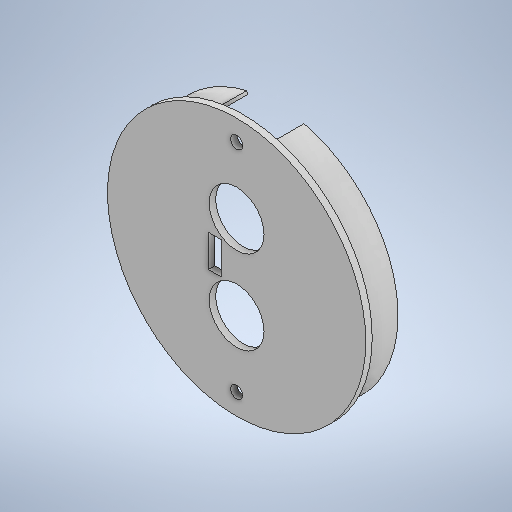
# Autodesk Inventor part: lid
Saved by Autodesk Inventor 2025.3 (Build 293356000, 356)
## iProperties
Created: 2025-04-18
Part Number: lid
Material: Generic
Document SubType Name: Modeling
Designer: Owner
Density: 1 g/cm^3
Appearance: Default
Author: Owner
Autodesk Inventor part; units mm, degrees
ref_plane "YZ Plane" through (0, 0, 0) normal (1, 0, 0) x (0, 1, 0)
ref_plane "XZ Plane" through (0, 0, 0) normal (0, 1, 0) x (-1, 0, 0)
ref_plane "XY Plane" through (0, 0, 0) normal (0, 0, 1) x (1, 0, 0)
sketch "Sketch1" plane through (0, 0, 0) normal (0, 0, 1) x (1, 0, 0)
  arc A0 (8.8755, -70.449) -> (8.8755, 3.449) centre (0, -33.5) ccw projected
  arc A1 (-8.8755, 3.449) -> (-8.8755, -70.449) centre (0, -33.5) ccw projected
  arc A2 (-8.6419, 2.4766) -> (-8.6419, -69.4766) centre (0, -33.5) ccw
  arc A3 (8.6419, -69.4766) -> (8.6419, 2.4766) centre (0, -33.5) ccw
  line L0 (-8.8755, 3.449) -> (-8.6419, 2.4766)
  line L1 (8.8755, 3.449) -> (8.6419, 2.4766)
  line L2 (-8.6419, -69.4766) -> (-8.8755, -70.449)
  line L3 (8.6419, -69.4766) -> (8.8755, -70.449)
  point P0 (0, 0)
  dimension "d0" = 1
  dimension "d1" = 1
  constraints: 8 end point, 4 point on circle, 2 centre point, 2 collinear
  measures "d0" radial gap between concentric circles of A1 A2
  measures "d1" radial gap between concentric circles of A0 A3
extrude "Extrusion1" add sketch "Sketch1" against normal blind 10
ref_plane "Work Plane1" through (0, 0, 0) normal (0, 0, 1) x (1, 0, 0)
sketch "Sketch2" plane through (0, 0, 0) normal (0, 0, 1) x (1, 0, 0)
  circle A0 centre (0, -33.5) radius 40 projected
  circle A1 centre (0, 0) radius 1.5 projected
  circle A2 centre (0, -67) radius 1.5 projected
  point P0 (0, 0)
extrude "Extrusion2" add sketch "Sketch2" along normal blind 2 contours A0 | A1 | A2
sketch "Sketch3" plane through (0, -33.5, 2) normal (0, 0, 1) x (1, 0, 0)
  circle A0 centre (0, 33.5) radius 1.875
  circle A1 centre (0, 33.5) radius 1.5 projected
  circle A2 centre (0, -33.5) radius 1.5 projected
  circle A3 centre (0, -33.5) radius 1.875
  dimension "d6" = 3.75
  dimension "d7" = 3.75
  constraints: 2 centre point, 2 coincident
  measures "d6" diameter of A0
  measures "d7" diameter of A3
extrude "Extrusion3" cut sketch "Sketch3" against normal up to surface (2 mm away) contours A0 | A1 | A2 | A3
sketch "Sketch4" plane through (0, -33.5, 2) normal (0, 0, 1) x (1, 0, 0)
  line L0 (-10, -22.5) -> (10, -22.5)
  line L1 (10, -22.5) -> (10, 22.5)
  line L2 (10, 22.5) -> (-10, 22.5)
  line L3 (-10, 22.5) -> (-10, -22.5)
  line L4 (-10, -22.5) -> (10, 22.5) construction
  line L5 (10, -22.5) -> (-10, 22.5) construction
  circle A0 centre (0, 13) radius 8.5
  circle A1 centre (0, -13) radius 8.5
  line L6 (-8.75, -5) -> (-4.75, -5)
  line L7 (-4.75, -5) -> (-4.75, 5)
  line L8 (-4.75, 5) -> (-8.75, 5)
  line L9 (-8.75, 5) -> (-8.75, -5)
  line L10 (-8.75, -5) -> (-4.75, 5) construction
  line L11 (-4.75, -5) -> (-8.75, 5) construction
  point P0 (0, 33.5)
  point P1 (0, 0)
  point P2 (-6.75, 0)
  dimension "d10" = 20
  dimension "d11" = 45
  dimension "d12" = 17
  dimension "d13" = 17
  dimension "d14" = 26
  dimension "d15" = 13
  dimension "d16" = 4
  dimension "d17" = 10
  dimension "d18" = 8.75
  constraints: 24 end point, 4 midpoint, 4 parallel, 2 centre point, 2 horizontal, 2 perpendicular
  measures "d10" distance of L2.end L1.end
  measures "d11" distance of L1.end L0.end
  measures "d12" diameter of A0
  measures "d13" diameter of A1
  measures "d14" distance of A1.centre A0.centre
  measures "d15" distance of point (0, 0) A1.centre
  measures "d16" distance of L8.end L7.end
  measures "d17" distance of L7.end L6.end
  measures "d18" distance from line of point (0, 0) L9
extrude "Extrusion4" cut sketch "Sketch4" against normal up to surface (2 mm away) contours A0 | A1 | L9 L8 L7 L6
body "Solid1"
